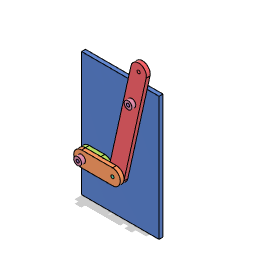
13. 揺動クランク（完成版） (Autodesk Fusion 360 design; units mm, degrees)
Autodesk Fusion 360 part; units mm, degrees
sketch "スケッチ1" plane through (0, 0, 0) normal (0, 0, 1) x (1, 0, 0)
  line L0 (40, 0) -> (90, 0)
  line L1 (90, 0) -> (90, 80)
  line L2 (90, 80) -> (40, 80)
  line L3 (40, 80) -> (40, 0)
  circle A0 centre (75, 70) radius 1
  line L4 (75, 70) -> (65, 25) construction
  line L5 (65, 25) -> (85, 25) construction
  line L6 (85, 25) -> (75, 70) construction
  circle A1 centre (55, 25) radius 1
  line L7 (125.1191, 71.0847) -> (115.1191, 26.0847)
  arc A2 (115.1191, 26.0847) -> (124.8809, 23.9153) centre (120, 25) ccw
  line L8 (124.8809, 23.9153) -> (134.8809, 68.9153)
  line L9 (130, 70) -> (120, 25) construction
  circle A3 centre (130, 70) radius 1
  circle A4 centre (120, 25) radius 1
  line L10 (5, 0) -> (5, 20)
  arc A5 (5, 20) -> (-5, 20) centre (0, 20) ccw
  line L11 (-5, 20) -> (-5, 0)
  arc A6 (-5, 0) -> (5, 0) centre (0, 0) ccw
  line L12 (0, 0) -> (0, 20) construction
  line L13 (20, 0) -> (20, 10)
  arc A7 (20, 10) -> (10, 10) centre (15, 10) ccw
  line L14 (10, 10) -> (10, 0)
  arc A8 (10, 0) -> (20, 0) centre (15, 0) ccw
  line L15 (15, 0) -> (15, 10) construction
  circle A9 centre (15, 10) radius 1
  circle A10 centre (15, 0) radius 1
  circle A11 centre (0, 20) radius 1
  circle A12 centre (0, 0) radius 1
  circle A13 centre (0, 50) radius 15
  circle A14 centre (0, 75) radius 1
  circle A15 centre (5, 75) radius 1
  circle A16 centre (10, 75) radius 1
  circle A17 centre (0, 50) radius 1
  circle A18 centre (5, 70) radius 1
  circle A19 centre (5, 70) radius 2.5
  line L16 (125.1191, 71.0847) -> (129.4577, 90.6084)
  line L17 (134.8809, 68.9153) -> (139.2195, 88.4391)
  arc A20 (139.2195, 88.4391) -> (129.4577, 90.6084) centre (134.3386, 89.5237) ccw
  circle A21 centre (134.3386, 89.5237) radius 1
  dimension "d1" = 2
  dimension "d3" = 2
  dimension "d4" = 10
  dimension "d5" = 20
  dimension "d6" = 10
  dimension "d7" = 10
  dimension "d8" = 2
  dimension "d9" = 2
  dimension "d10" = 2
  dimension "d11" = 2
  dimension "d12" = 30
  dimension "d13" = 2
  dimension "d14" = 2
  dimension "d15" = 2
  dimension "d18" = 2
  dimension "d39" = 5
  dimension "d100" = 20
  dimension "d101" = 20
  dimension "d102" = 2
  constraint horizontal L0
  constraint vertical L1
  constraint horizontal L2
  constraint vertical L3
  constraint coincident A0.centre L4.start
  constraint perpendicular L1 L5
  constraint tangent L7 A2
  constraint tangent A2 L8
  constraint parallel L7 L8
  constraint concentric A2 A4
  constraint tangent L10 A5
  constraint tangent A5 L11
  constraint parallel L10 L11
  constraint tangent L11 A6
  constraint tangent L10 A6
  constraint vertical L12
  constraint coincident A6.centre L12.start
  constraint tangent L13 A7
  constraint tangent A7 L14
  constraint parallel L13 L14
  constraint tangent L14 A8
  constraint tangent L13 A8
  constraint vertical L15
  constraint concentric A7 A9
  constraint concentric A8 A10
  constraint concentric A5 A11
  constraint concentric A6 A12
  constraint concentric A13 A17
  constraint concentric A18 A19
  constraint tangent L17 A20
  constraint concentric A20 A21
  measures "d1" diameter of A0
  measures "d3" diameter of A1
  measures "d4" diameter of A2
  measures "d5" distance of A6.centre A5.centre
  measures "d6" diameter of A5
  measures "d7" diameter of A7
  measures "d8" diameter of A9
  measures "d9" diameter of A10
  measures "d10" diameter of A11
  measures "d11" diameter of A12
  measures "d12" diameter of A13
  measures "d13" diameter of A14
  measures "d14" diameter of A15
  measures "d15" diameter of A16
  measures "d18" diameter of A17
  measures "d39" diameter of A19
  measures "d100" distance of L7.start L16.end
  measures "d101" distance of L8.end L17.end
  measures "d102" diameter of A21
extrude "押し出し1" add sketch "スケッチ1" along normal blind 2.5 contours L0 L1 L2 L3 | L7 A2 L8 L16 L17 A20 | L10 A5 L11 A6 | L13 A7 L14 A8 makes body 1 at (11.4588, 6.4061, 0) makes body 2 at (-3.4551, 13.023, 0) makes body 3 at (73.7927, 31.4887, 0) makes body 4 at (125.1323, 39.5982, 0)
extrude "押し出し2" add sketch "スケッチ1" along normal blind 15 separate body contours A13 makes body 5
extrude "押し出し3" add sketch "スケッチ1" along normal blind 5 contours A17 bodies 5
extrude "押し出し1'" add sketch "スケッチ1" along normal blind 15 separate body contours A14 makes body 6 in component "軸1"
copy_body "ボディ -> コンポーネント1" bodies 5 removing the originals makes body 7 in component "ノブ"
copy_body "ボディ -> コンポーネント2" bodies 1 removing the originals makes body 8 in component "リンク1"
copy_body "ボディ -> コンポーネント3" bodies 2 removing the originals makes body 9 in component "リンク2"
copy_body "ボディ -> コンポーネント4" bodies 3 removing the originals makes body 10 in component "側面"
copy_body "ボディ -> コンポーネント5" bodies 4 removing the originals makes body 11 in component "従動節"
extrude "押し出し1''" add sketch "スケッチ1" along normal blind 7.5 separate body contours A15 makes body 12 in component "軸2"
extrude "押し出し1'''" add sketch "スケッチ1" along normal blind 2.5 separate body contours A19 makes body 13 in component "留め具"
extrude "押し出し1''''" add sketch "スケッチ1" along normal blind 5 separate body contours A15 makes body 14 in component "軸3"
component "従動節" placed x (1, 0, 0) y (0, 1, 0) z (0, 0, 1) at (-55, 0, 2.5)
component "軸3" placed x (0, 1, 0) y (-1, 0, 0) z (0, 0, 1) at (140, 20, 2.5)
component "リンク2" placed x (0, 1, 0) y (-1, 0, 0) z (0, 0, 1) at (65, 25, 5)
component "軸2" placed x (0, -1, 0) y (1, 0, 0) z (0, 0, 1) at (-30, 30, 2.5)
component "留め具" placed x (0, -1, 0) y (1, 0, 0) z (0, 0, 1) at (-25, 30, 7.5)
component "リンク1" placed x (0, -1, 0) y (1, 0, 0) z (0, 0, 1) at (45, 40, 2.5)
component "軸1" placed x (0, -1, 0) y (1, 0, 0) z (0, 0, 1) at (-20, 25, -10)
component "ノブ" placed x (0, -1, 0) y (1, 0, 0) z (0, 0, 1) at (5, 25, -15)
component "留め具" placed x (1, 0, 0) y (0, 1, 0) z (0, 0, 1) at (70, 0, 5)
component "軸2" placed x (1, 0, 0) y (0, 1, 0) z (0, 0, 1) at (70, -5, 0)
component "側面" placed x (1, 0, 0) y (0, 1, 0) z (0, 0, 1) at (0, 0, 0)
named bodies: "リンク1", "リンク2", "側面", "リンク3"
